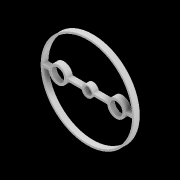
# Autodesk Inventor part: Magnet_rotor_parametriserad_02
Saved by Autodesk Inventor 2020 (Build 240168000, 168)
## iProperties
Created: 2020-11-21
Part Number: Magnet_rotor_parametriserad_02
Material: Generic
Document SubType Name: Modeling
Designer: Gottfrid
Density: 1 g/cm^3
Appearance: Default
D_axel: 7.000 mm
d_axelRing: 3.000 mm
r_filletAxel: 0,400 mm
D_yttreRing_i: 80.000 mm
d_yttreRing: 3.000 mm
d_stöttor: 1.800 mm
Author: Gottfrid
Autodesk Inventor part; units mm, degrees
ref_plane "YZ Plane" through (0, 0, 0) normal (1, 0, 0) x (0, 1, 0)
ref_plane "XZ Plane" through (0, 0, 0) normal (0, 1, 0) x (-1, 0, 0)
ref_plane "XY Plane" through (0, 0, 0) normal (0, 0, 1) x (1, 0, 0)
sketch "Sketch1" plane through (0, 0, 0) normal (0, 0, 1) x (1, 0, 0)
  circle A0 centre (0, 0) radius 40
  circle A1 centre (0, 0) radius 41.5
  circle A2 centre (0, 0) radius 3.5
  circle A3 centre (0, 0) radius 5
  circle A4 centre (26, 0) radius 6.8
  circle A5 centre (26, 0) radius 7.8
  line L0 (0, 0) -> (43.8957, 0) construction
  line L1 (4.9183, 0.9) -> (18.2521, 0.9)
  line L2 (33.7479, 0.9) -> (39.9899, 0.9)
  line L3 (4.9183, -0.9) -> (18.2521, -0.9)
  line L4 (33.7479, -0.9) -> (39.9899, -0.9)
  line L5 (-4.9183, -0.9) -> (-18.2521, -0.9)
  line L6 (-4.9183, 0.9) -> (-18.2521, 0.9)
  circle A6 centre (-26, 0) radius 7.8
  circle A7 centre (-26, 0) radius 6.8
  line L7 (-33.7479, 0.9) -> (-39.9899, 0.9)
  line L8 (-33.7479, -0.9) -> (-39.9899, -0.9)
  line L9 (1.2333, -3.7857) -> (-1.2333, -3.7857)
  line L10 (-1.6333, -3.3857) -> (-1.6333, 3.3857)
  line L11 (-1.2333, 3.7857) -> (1.2333, 3.7857)
  line L12 (1.6333, 3.3857) -> (1.6333, -3.3857)
  line L13 (1.6333, -3.7857) -> (-1.6333, 3.7857) construction
  line L14 (-1.6333, -3.7857) -> (1.6333, 3.7857) construction
  arc A8 (-1.2333, 3.7857) -> (-1.6333, 3.3857) centre (-1.2333, 3.3857) ccw
  arc A9 (1.6333, 3.3857) -> (1.2333, 3.7857) centre (1.2333, 3.3857) ccw
  arc A10 (1.2333, -3.7857) -> (1.6333, -3.3857) centre (1.2333, -3.3857) ccw
  arc A11 (-1.6333, -3.3857) -> (-1.2333, -3.7857) centre (-1.2333, -3.3857) ccw
  line L15 (3.3857, -1.6333) -> (-3.3857, -1.6333)
  line L16 (-3.7857, -1.2333) -> (-3.7857, 1.2333)
  line L17 (-3.3857, 1.6333) -> (3.3857, 1.6333)
  line L18 (3.7857, 1.2333) -> (3.7857, -1.2333)
  line L19 (3.7857, -1.6333) -> (-3.7857, 1.6333) construction
  line L20 (-3.7857, -1.6333) -> (3.7857, 1.6333) construction
  arc A12 (-3.3857, 1.6333) -> (-3.7857, 1.2333) centre (-3.3857, 1.2333) ccw
  arc A13 (3.7857, 1.2333) -> (3.3857, 1.6333) centre (3.3857, 1.2333) ccw
  arc A14 (3.3857, -1.6333) -> (3.7857, -1.2333) centre (3.3857, -1.2333) ccw
  arc A15 (-3.7857, -1.2333) -> (-3.3857, -1.6333) centre (-3.3857, -1.2333) ccw
  point P0 (-4.9183, -0.9)
  point P1 (4.9183, -0.9)
  point P2 (-1.6333, -3.0955)
  point P3 (-1.6333, 3.0955)
  point P4 (1.6333, 3.0955)
  point P5 (1.6333, -3.0955)
  point P6 (-4.9183, 0.9)
  point P7 (-33.7479, 0.9)
  point P8 (-3.0955, -1.6333)
  point P9 (-3.0955, 1.6333)
  point P10 (3.0955, 1.6333)
  point P11 (3.0955, -1.6333)
  dimension "d0" = 80
  dimension "d3" = 10
  dimension "d1" = 83
  dimension "d2" = 7
  dimension "d4" = 13.6
  dimension "d5" = 26
  dimension "d6" = 15.6
  dimension "d10" = 0.9
  dimension "d11" = 0.9
  dimension "d14" = 360
  dimension "d16" = 7.5714
  dimension "d17" = 3.2667
  dimension "d18" = 0.4
  dimension "d29" = 7.5714
  dimension "d30" = 3.2667
  dimension "d31" = 0.4
  constraints: 42 end point, 20 point on circle, 16 point on line, 16 tangent, 14 centre point, 8 coincident, 6 equal radius, 5 horizontal, 4 midpoint, 4 parallel, 4 symmetric about line, 2 perpendicular, 1 horizontal alignment, 39 other
  measures "d1" diameter of A1
  measures "d2" diameter of A2
  measures "d4" diameter of A4
  measures "d5" distance of A4.centre point (0, 0)
  measures "d6" diameter of A5
  measures "d10" vertical distance of L1.start point (0, 0)
  measures "d11" distance between parallel lines of L0 L2
  measures "d16" distance between parallel lines of L9 L11
  measures "d17" distance between parallel lines of L12 L10
  measures "d18" radius of A8
  measures "d29" distance between parallel lines of L18 L16
  measures "d30" distance between parallel lines of L15 L17
  measures "d31" radius of A12
extrude "Extrusion1" add sketch "Sketch1" along normal blind 5 contours A0 L4 A5 L2 | L7 A6 L8 A0 | A5 | A6 | A5 L3 A3 L1 | L6 A3 L5 A6 | A3 | A1
sketch "Sketch2" plane through (0, 0, 5) normal (0, 0, 1) x (1, 0, 0)
  arc A0 (33.7479, 0.9) -> (18.2521, 0.9) centre (26, 0) ccw projected
  circle A1 centre (26, 0) radius 7.7
  circle A2 centre (26, 0) radius 5.8
  arc A3 (18.2521, -0.9) -> (33.7479, -0.9) centre (26, 0) ccw projected
  circle A4 centre (-26, 0) radius 5.8
  circle A5 centre (-26, 0) radius 7.7
  point P0 (0, 0)
  point P1 (18.3528, 0.9)
  point P2 (33.6472, 0.9)
  point P3 (-18.2521, 0.9)
  point P4 (-33.7479, 0.9)
  point P5 (18.7723, -2.9327)
  dimension "d21" = 7.8
  dimension "d22" = 11.6
  dimension "d27" = 360
  constraints: 2 centre point, 2 coincident, 1 concentric, 17 other
  measures "d21" radius of A0
  measures "d22" diameter of A2
extrude "Extrusion2" add sketch "Sketch2" along normal blind 0.4
equation "\"d0\" = D_yttreRing_i"
equation "\"d3\" = D_axel + d_axelRing"
equation "\"d1\" = D_yttreRing_i + d_yttreRing"
equation "\"d2\" = D_axel"
equation "\"d4\" = D_magnet + d_toleransRing"
equation "\"d5\" = l_magnetHållarRingFrånOrigo"
equation "\"d6\" = d_toleransRing + D_magnet + d_magnetHållarRing"
equation "\"d10\" = 0.5 * d_stöttor"
equation "\"d11\" = 0.5 * d_stöttor"
equation "\"d18\" = r_filletAxel"
equation "\"d31\" = r_filletAxel"
equation "\"d19\" = h_höjdMagnetRotor"
equation "\"d22\" = D_magnet - d_magnetSkydd"
equation "\"d23\" = h_magnetSkydd"
equation "\"D_yttreRing_i\" = 80"
equation "\"d_yttreRing\" = 3"
equation "\"D_magnet\" = 13"
equation "\"D_axel\" = 7"
equation "\"d_axelRing\" = 3"
equation "\"h_höjdMagnetRotor\" = 5"
equation "\"d_stöttor\" = 1.8"
equation "\"d_toleransRing\" = 0.6"
equation "\"d_magnetHållarRing\" = 2"
equation "\"l_magnetHållarRingFrånOrigo\" = 26"
equation "\"r_filletAxel\" = 0.4"
equation "\"h_magnetSkydd\" = 0.4"
equation "\"d_magnetSkydd\" = 1.4"
body "Solid1"
